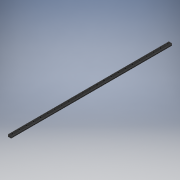
# Autodesk Inventor part: SSE2B-MX10-455_r
Saved by Autodesk Inventor 2019 (Build 230136000, 136)
## iProperties
Created: 2024-08-09
Part Number: SSE2B-MX10-455_r
Material: Generic
Catalog Web Link: www.cadenas.de
Description: SSEB, SSEB-MX, SSEBV, SSEBV-MX, SSE2B, SSE2B-MX, SSE2BV, SSE2BV-MX, SSEBL, SSEBL-MX, SSEBLV, SSEBLV-MX, SSE2BL, SSE2BL-MX, SSE2BLV, SSE2BLV-MX, SEB, SEBV, SE2B, SE2BV, SEBL, SEBLV, SE2BL, SE2BLV_rail-Miniature Linear Guides - Short Block, Standard Preload - High/Precision Grade
Vendor: MISUMI
Document SubType Name: Modeling
Designer: psAdmin
Manufacturer: MISUMI
Mass: 18.2654 g
Surface Area: 164.286 cm^2
Volume: 18.2654 cm^3
Density: 1 g/cm^3
Appearance: PSOLRGB-175-175-175
Category: PARTsolutions
Company: MISUMI
Title: SSE2B-MX10-455
Author: Cadenas PARTsolutions
Comments: Miniature Linear Guides - Short Block, Standard Preload - High/Precision Grade
PSOL_IDENT_0: {$CADENAS_DATA/23d-libs/misumi/metric/06_linear_guides/seb_series/seb_rail.prj},403 {VTYP=3D},{NB=SS
PSOL_IDENT_1: E2B-MX10-455_r},{LINA=SSE2B-MX10-455},{NN=SSEB, SSEB-MX, SSEBV, SSEBV-MX, SSE2B, SSE2B-MX, SSE2BV, S
PSOL_IDENT_2: SE2BV-MX, SSEBL, SSEBL-MX, SSEBLV, SSEBLV-MX, SSE2BL, SSE2BL-MX, SSE2BLV, SSE2BLV-MX, SEB, SEBV, SE2
PSOL_IDENT_3: B, SE2BV, SEBL, SEBLV, SE2BL, SE2BLV_rail},{DATE=17.02.2022 00:32:34},{GEOMDATE=21.01.2022 00:02:30}
PSOL_IDENT_4: ,{VERSION=},{LINEID=160},{WBVAR=TS,ST,MAT,MX,NOB,LT,LS,ALT1,ALT2,ALT4},{WBNUMERIC=LS}  {NB=SSE2B-MX1
PSOL_IDENT_5: 0-455_r},{LINA=SSE2B-MX10-455},{KT=DUMMY},{PN=SSE2B-MX10-455},{RT=B},{TS=},{TS1=  '','Advanced','V','
PSOL_IDENT_6: Precision'  },{TYPE=SSE2B},{ST=S},{MAT=S},{MX=-MX},{MXALG='', 'w/o MX(Lubrication unit)', '-MX', 'wi
PSOL_IDENT_7: th MX(Lubrication unit)'},{NOB=2},{H=10},{LT=Selectable},{LTALG='Selectable','Selectable','Configura
PSOL_IDENT_8: ble','Configurable'},{LS=455},{W=20},{L1=30.0},{B=15},{C=10},{S=M3x3},{L2=19.0},{K=7.8},{CBB=0.3},{W
PSOL_IDENT_9: 1=9},{W2=5.5},{H1=5.5},{CAA=0.3},{DD1DD2HH=3.5x6x3.5},{F=20},{G=7.5},{DD1=3.500},{DD2=6.000},{HH=3.5
PSOL_IDENT_10: 00},{ALT1=},{ALT1ALG='', 'Not applicable'},{MC=M4},{MC1=4.0},{ALT2=},{ALT2L=2.5},{ALT2N=5},{M=23},{L
PSOL_IDENT_11: L=},{L0=75,95,115,135,155,175,195,215,235,255,275,295,315,335,355,355,375,395,415,435,455,475,495,51
PSOL_IDENT_12: 5,535,555,575,595,615,635},{REC1=   '','w/o Rail Ends Cut alteration','-LLC','with LLC (Left End Cut
PSOL_IDENT_13: )','-RLC','with RLC (Right End Cut)','-LLC-RLC','with Both End Cut'   },{ST1='S', 'w/o Surface Treat
PSOL_IDENT_14: ment','R','Low Temperature Black Chrome Plating'},{MAT2= 'S','Stainless Steel','','Carbon Steel' },{
PSOL_IDENT_15: NL=113.750},{ALT4=},{ALT4ALG= '','N/A' },{CA1=0.2},{CA2=0.3},{VA1=1.5},{HA1=1.4},{HA2=9.5430},{WA1=2
PSOL_IDENT_16: .0868},{WA2=0.7},{RA1=2.20},{POIA1=0.1400},{NA1=22},{LSC=0.0},{MS=0.0}
NB: SSE2B-MX10-455_r
NN: SSEB, SSEB-MX, SSEBV, SSEBV-MX, SSE2B, SSE2B-MX, SSE2BV, SSE2BV-MX, SSEBL, SSEBL-MX, SSEBLV, SSEBLV-MX, SSE2BL, SSE2BL-MX, SSE2BLV, SSE2BLV-MX, SEB, SEBV, SE2B, SE2BV, SEBL, SEBLV, SE2BL, SE2BLV_rail
NT: Miniature Linear Guides - Short Block, Standard Preload - High/Precision Grade
NBSYN: $PN._r
LINA: SSE2B-MX10-455
CATALOG: Misumi
PN: SSE2B-MX10-455
TS: Advanced
ST: w/o Surface Treatment
MAT: Stainless Steel
MX: with MX(Lubrication unit)
NOB: 2
H: 10
LT: Selectable
LS: 455
W: 20
L1: 30
B: 15
C: 10
S: M3x3
L2: 19
K: 7.8
CBB: 0.3
W1: 9
W2: 5.5
H1: 5.5
CAA: 0.3
DD1DD2HH: 3.5x6x3.5
F: 20
G: 7.5
ALT1: Not applicable
ALT2: w/o Rail Ends Cut alteration
ALT4: N/A
NA1: 22
SUPPLIER: MISUMI
ARTICLENO: SSE2B-MX10-455_r
BOMINFO: SSE2B-MX10-455
CREATOR: CADENAS GmbH
Autodesk Inventor part; units mm, degrees
sketch "Sketch_12" plane through (0, 0, 0) normal (0, 0, 1) x (1, 0, 0)
  line L0 (-4.5, 5.3) -> (-4.5, 5.0434)
  line L1 (-4.5, 5.0434) -> (-4.2216, 4.8827)
  arc A0 (-3.7548, 4.35) -> (-4.2216, 4.8827) centre (-4.7715, 3.93) ccw
  line L2 (-3.7548, 4.35) -> (-3.1, 4.35)
  line L3 (-3.1, 4.35) -> (-3.1, 3.65)
  line L4 (-3.1, 3.65) -> (-3.7548, 3.65)
  arc A1 (-4.2216, 3.1173) -> (-3.7548, 3.65) centre (-4.7715, 4.07) ccw
  line L5 (-4.2216, 3.1173) -> (-4.5, 2.9566)
  line L6 (-4.5, 2.9566) -> (-4.5, 0.3)
  line L7 (-4.5, 0.3) -> (-4.2, 0)
  line L8 (-4.2, 0) -> (4.2, 0)
  line L9 (4.2, 0) -> (4.5, 0.3)
  line L10 (4.5, 0.3) -> (4.5, 2.9566)
  line L11 (4.5, 2.9566) -> (4.2216, 3.1173)
  arc A2 (3.7548, 3.65) -> (4.2216, 3.1173) centre (4.7715, 4.07) ccw
  line L12 (3.7548, 3.65) -> (3.1, 3.65)
  line L13 (3.1, 3.65) -> (3.1, 4.35)
  line L14 (3.1, 4.35) -> (3.7548, 4.35)
  arc A3 (4.2216, 4.8827) -> (3.7548, 4.35) centre (4.7715, 3.93) ccw
  line L15 (4.2216, 4.8827) -> (4.5, 5.0434)
  line L16 (4.5, 5.0434) -> (4.5, 5.3)
  line L17 (4.5, 5.3) -> (4.3, 5.5)
  line L18 (4.3, 5.5) -> (-4.3, 5.5)
  line L19 (-4.3, 5.5) -> (-4.5, 5.3)
  constraints: 40 end point, 8 point on circle, 4 centre point
extrude "Extrusion1" add sketch "Sketch_12" along normal mid plane 455
sketch "Sketch2" plane through (-4.3, 5.5, 227.5) normal (0, 1, 0) x (1, 0, 0)
  point P0 (4.3, 447.5)
hole "Hole1" at (0, 5.5, -220) direction (0, -1, 0) diameter 3.5 depth 5.5 counterbore diameter 6 counterbore depth 3.5
pattern_linear "Rectangular Pattern1" count 23 spacing 20 along (0, 0, 1) of "Hole1"
ref_plane "rail_to_adjusting_block_XY" through (0, 0, -220) normal (0, 1, 0) x (1, 0, 0)
ref_plane "rail_to_adjusting_block_YZ" through (0, 0, -220) normal (1, 0, 0) x (0, 0, -1)
ref_plane "rail_to_adjusting_block_ZX" through (0, 0, -220) normal (0, 0, -1) x (0, 1, 0)
ref_plane "to_block_XY" through (0, 5.5, 113.75) normal (0, 0, 1) x (1, 0, 0)
ref_plane "to_block_YZ" through (0, 5.5, 113.75) normal (1, 0, 0) x (0, 1, 0)
ref_plane "to_block_ZX" through (0, 5.5, 113.75) normal (0, 1, 0) x (0, 0, 1)
ref_plane "to_block_2_XY" through (0, 5.5, -113.75) normal (0, 0, 1) x (1, 0, 0)
ref_plane "to_block_2_YZ" through (0, 5.5, -113.75) normal (1, 0, 0) x (0, 1, 0)
ref_plane "to_block_2_ZX" through (0, 5.5, -113.75) normal (0, 1, 0) x (0, 0, 1)
ref_plane "to_kue_XY" through (0, 0, 0) normal (0, 1, 0) x (1, 0, 0)
ref_plane "to_kue_YZ" through (0, 0, 0) normal (1, 0, 0) x (0, 0, -1)
ref_plane "to_kue_ZX" through (0, 0, 0) normal (0, 0, -1) x (0, 1, 0)
body "Solid1"
